Autodesk Fusion 360 part; units mm, degrees
(part 7 of 40)
  line L2812 (187.5144, 92.3152) -> (187.4885, 92.1609) construction
  line L2813 (187.4885, 92.1609) -> (187.4646, 92.006) construction
  line L2814 (187.4646, 92.006) -> (187.4423, 91.8506) construction
  line L2815 (187.4423, 91.8506) -> (187.4215, 91.6948) construction
  line L2816 (187.4215, 91.6948) -> (187.4019, 91.5386) construction
  line L2817 (187.4019, 91.5386) -> (187.3835, 91.3821) construction
  line L2818 (187.3835, 91.3821) -> (187.3662, 91.2253) construction
  line L2819 (187.3662, 91.2253) -> (187.3502, 91.0682) construction
  line L2820 (187.3502, 91.0682) -> (187.3355, 90.9107) construction
  line L2821 (187.3355, 90.9107) -> (187.3222, 90.7529) construction
  line L2822 (187.3222, 90.7529) -> (187.3102, 90.5947) construction
  line L2823 (187.3102, 90.5947) -> (187.2995, 90.4362) construction
  line L2824 (187.2995, 90.4362) -> (187.29, 90.2774) construction
  line L2825 (187.29, 90.2774) -> (187.2816, 90.1183) construction
  line L2826 (187.2816, 90.1183) -> (187.2743, 89.9589) construction
  line L2827 (187.2743, 89.9589) -> (187.2682, 89.7993) construction
  line L2828 (187.2682, 89.7993) -> (187.2631, 89.6395) construction
  line L2829 (187.2631, 89.6395) -> (187.2591, 89.4794) construction
  line L2830 (187.2591, 89.4794) -> (187.2563, 89.3191) construction
  line L2831 (187.2563, 89.3191) -> (187.2544, 89.1585) construction
  line L2832 (187.2544, 89.1585) -> (187.2537, 88.9977) construction
  line L2833 (187.2537, 88.9977) -> (187.254, 88.8367) construction
  line L2834 (187.254, 88.8367) -> (187.2554, 88.6755) construction
  line L2835 (187.2554, 88.6755) -> (187.2578, 88.5141) construction
  line L2836 (187.2578, 88.5141) -> (187.2612, 88.3525) construction
  line L2837 (187.2612, 88.3525) -> (187.2655, 88.1907) construction
  line L2838 (187.2655, 88.1907) -> (187.2709, 88.0288) construction
  line L2839 (187.2709, 88.0288) -> (187.2772, 87.8666) construction
  line L2840 (187.2772, 87.8666) -> (187.2845, 87.7043) construction
  line L2841 (187.2845, 87.7043) -> (187.2928, 87.5419) construction
  line L2842 (187.2928, 87.5419) -> (187.302, 87.3793) construction
  line L2843 (187.302, 87.3793) -> (187.3121, 87.2165) construction
  line L2844 (187.3121, 87.2165) -> (187.3232, 87.0536) construction
  line L2845 (187.3232, 87.0536) -> (187.3353, 86.8905) construction
  line L2846 (187.3353, 86.8905) -> (187.3482, 86.7273) construction
  line L2847 (187.3482, 86.7273) -> (187.362, 86.564) construction
  line L2848 (187.362, 86.564) -> (187.3768, 86.4005) construction
  line L2849 (187.3768, 86.4005) -> (187.3924, 86.2369) construction
  line L2850 (187.3924, 86.2369) -> (187.409, 86.0732) construction
  line L2851 (187.409, 86.0732) -> (187.4264, 85.9094) construction
  line L2852 (187.4264, 85.9094) -> (187.4447, 85.7455) construction
  line L2853 (187.4447, 85.7455) -> (187.4639, 85.5815) construction
  line L2854 (187.4639, 85.5815) -> (187.484, 85.4174) construction
  line L2855 (187.484, 85.4174) -> (187.5049, 85.2532) construction
  line L2856 (187.5049, 85.2532) -> (187.5266, 85.0889) construction
  line L2857 (187.5266, 85.0889) -> (187.5492, 84.9245) construction
  line L2858 (187.5492, 84.9245) -> (187.5727, 84.76) construction
  line L2859 (187.5727, 84.76) -> (187.597, 84.5954) construction
  line L2860 (187.597, 84.5954) -> (187.6222, 84.4308) construction
  line L2861 (187.6222, 84.4308) -> (187.6481, 84.266) construction
  line L2862 (187.6481, 84.266) -> (187.6749, 84.1013) construction
  line L2863 (187.6749, 84.1013) -> (187.7026, 83.9364) construction
  line L2864 (187.7026, 83.9364) -> (187.731, 83.7715) construction
  line L2865 (187.731, 83.7715) -> (187.7602, 83.6065) construction
  line L2866 (187.7602, 83.6065) -> (187.7903, 83.4415) construction
  line L2867 (187.7903, 83.4415) -> (187.8212, 83.2764) construction
  line L2868 (187.8212, 83.2764) -> (187.8528, 83.1113) construction
  line L2869 (187.8528, 83.1113) -> (187.8788, 82.9792) construction
  line L2870 (187.8788, 82.9792) -> (187.8986, 82.8801) construction
  line L2871 (187.8986, 82.8801) -> (187.912, 82.814) construction
  line L2872 (187.912, 82.814) -> (187.9188, 82.7809) construction
  arc A97 (187.9188, 82.7809) -> (192.2105, 81.3864) centre (212.132, 150) ccw
  arc A98 (187.9188, 82.7809) -> (192.2105, 81.3864) centre (212.132, 150) ccw
  line L2873 (256.7226, 110.7517) -> (257.9473, 109.6737)
  line L2874 (256.7226, 110.7517) -> (257.9473, 109.6737)
  arc A99 (269.1057, 157.2806) -> (268.567, 160.6816) centre (212.132, 150) ccw
  arc A100 (269.1057, 157.2806) -> (268.567, 160.6816) centre (212.132, 150) ccw
  arc A101 (256.7226, 110.7517) -> (253.9452, 110.6216) centre (255.4012, 109.2504) ccw
  arc A102 (256.7226, 110.7517) -> (253.9452, 110.6216) centre (255.4012, 109.2504) ccw
  arc A103 (251.5104, 108.1868) -> (253.9452, 110.6216) centre (212.132, 150) ccw
  arc A104 (251.5104, 108.1868) -> (253.9452, 110.6216) centre (212.132, 150) ccw
  spline S38 degree 5 poles (257.9473, 109.6737) (257.9705, 109.6533) (258.0174, 109.6132) (258.0893, 109.5549) (258.188, 109.4808) (258.3153, 109.3934) (258.4455, 109.3096) (258.5774, 109.228) (258.7102, 109.1476) (258.8437, 109.068) (258.9778, 108.9893) (259.1127, 108.9117) (259.2488, 108.8358) (259.3863, 108.7617) (259.525, 108.6894) (259.6649, 108.6187) (259.8058, 108.5496) (259.9476, 108.4816) (260.0901, 108.4147) (260.2332, 108.3488) (260.377, 108.284) (260.5215, 108.2202) (260.6667, 108.1576) (260.8127, 108.0961) (260.9594, 108.0358) (261.1069, 107.9766) (261.255, 107.9185) (261.4037, 107.8614) (261.553, 107.8053) (261.7029, 107.7501) (261.8534, 107.6959) (262.0044, 107.6426) (262.156, 107.5903) (262.3081, 107.539) (262.4608, 107.4886) (262.614, 107.4392) (262.7678, 107.3906) (262.922, 107.343) (263.0767, 107.2963) (263.2319, 107.2505) (263.3876, 107.2055) (263.5438, 107.1614) (263.7004, 107.1182) (263.8575, 107.0759) (264.015, 107.0344) (264.1729, 106.9937) (264.3313, 106.9539) (264.4901, 106.915) (264.6493, 106.8769) (264.8089, 106.8396) (264.9689, 106.8031) (265.1293, 106.7674) (265.2901, 106.7326) (265.4513, 106.6985) (265.6129, 106.6653) (265.7748, 106.6328) (265.9371, 106.6012) (266.0997, 106.5703) (266.2627, 106.5403) (266.426, 106.511) (266.5897, 106.4825) (266.7537, 106.4547) (266.9181, 106.4277) (267.0828, 106.4016) (267.2478, 106.3761) (267.4131, 106.3514) (267.5787, 106.3275) (267.7446, 106.3044) (267.9109, 106.282) (268.0774, 106.2603) (268.2442, 106.2394) (268.3779, 106.2233) (268.4783, 106.2115) (268.5453, 106.2038) (268.5789, 106.2) knots 0 0 0 0 0 0 0.01428571 0.02857143 0.04285714 0.05714286 0.07142857 0.08571429 0.1 0.11428571 0.12857143 0.14285714 0.15714286 0.17142857 0.18571429 0.2 0.21428571 0.22857143 0.24285714 0.25714286 0.27142857 0.28571429 0.3 0.31428571 0.32857143 0.34285714 0.35714286 0.37142857 0.38571429 0.4 0.41428571 0.42857143 0.44285714 0.45714286 0.47142857 0.48571429 0.5 0.51428571 0.52857143 0.54285714 0.55714286 0.57142857 0.58571429 0.6 0.61428571 0.62857143 0.64285714 0.65714286 0.67142857 0.68571429 0.7 0.71428571 0.72857143 0.74285714 0.75714286 0.77142857 0.78571429 0.8 0.81428571 0.82857143 0.84285714 0.85714286 0.87142857 0.88571429 0.9 0.91428571 0.92857143 0.94285714 0.95714286 0.97142857 0.98571429 1 1 1 1 1 1
  line L2875 (257.9473, 109.6737) -> (257.9705, 109.6533) construction
  line L2876 (257.9705, 109.6533) -> (258.0174, 109.6132) construction
  line L2877 (258.0174, 109.6132) -> (258.0893, 109.5549) construction
  line L2878 (258.0893, 109.5549) -> (258.188, 109.4808) construction
  line L2879 (258.188, 109.4808) -> (258.3153, 109.3934) construction
  line L2880 (258.3153, 109.3934) -> (258.4455, 109.3096) construction
  line L2881 (258.4455, 109.3096) -> (258.5774, 109.228) construction
  line L2882 (258.5774, 109.228) -> (258.7102, 109.1476) construction
  line L2883 (258.7102, 109.1476) -> (258.8437, 109.068) construction
  line L2884 (258.8437, 109.068) -> (258.9778, 108.9893) construction
  line L2885 (258.9778, 108.9893) -> (259.1127, 108.9117) construction
  line L2886 (259.1127, 108.9117) -> (259.2488, 108.8358) construction
  line L2887 (259.2488, 108.8358) -> (259.3863, 108.7617) construction
  line L2888 (259.3863, 108.7617) -> (259.525, 108.6894) construction
  line L2889 (259.525, 108.6894) -> (259.6649, 108.6187) construction
  line L2890 (259.6649, 108.6187) -> (259.8058, 108.5496) construction
  line L2891 (259.8058, 108.5496) -> (259.9476, 108.4816) construction
  line L2892 (259.9476, 108.4816) -> (260.0901, 108.4147) construction
  line L2893 (260.0901, 108.4147) -> (260.2332, 108.3488) construction
  line L2894 (260.2332, 108.3488) -> (260.377, 108.284) construction
  line L2895 (260.377, 108.284) -> (260.5215, 108.2202) construction
  line L2896 (260.5215, 108.2202) -> (260.6667, 108.1576) construction
  line L2897 (260.6667, 108.1576) -> (260.8127, 108.0961) construction
  line L2898 (260.8127, 108.0961) -> (260.9594, 108.0358) construction
  line L2899 (260.9594, 108.0358) -> (261.1069, 107.9766) construction
  line L2900 (261.1069, 107.9766) -> (261.255, 107.9185) construction
  line L2901 (261.255, 107.9185) -> (261.4037, 107.8614) construction
  line L2902 (261.4037, 107.8614) -> (261.553, 107.8053) construction
  line L2903 (261.553, 107.8053) -> (261.7029, 107.7501) construction
  line L2904 (261.7029, 107.7501) -> (261.8534, 107.6959) construction
  line L2905 (261.8534, 107.6959) -> (262.0044, 107.6426) construction
  line L2906 (262.0044, 107.6426) -> (262.156, 107.5903) construction
  line L2907 (262.156, 107.5903) -> (262.3081, 107.539) construction
  line L2908 (262.3081, 107.539) -> (262.4608, 107.4886) construction
  line L2909 (262.4608, 107.4886) -> (262.614, 107.4392) construction
  line L2910 (262.614, 107.4392) -> (262.7678, 107.3906) construction
  line L2911 (262.7678, 107.3906) -> (262.922, 107.343) construction
  line L2912 (262.922, 107.343) -> (263.0767, 107.2963) construction
  line L2913 (263.0767, 107.2963) -> (263.2319, 107.2505) construction
  line L2914 (263.2319, 107.2505) -> (263.3876, 107.2055) construction
  line L2915 (263.3876, 107.2055) -> (263.5438, 107.1614) construction
  line L2916 (263.5438, 107.1614) -> (263.7004, 107.1182) construction
  line L2917 (263.7004, 107.1182) -> (263.8575, 107.0759) construction
  line L2918 (263.8575, 107.0759) -> (264.015, 107.0344) construction
  line L2919 (264.015, 107.0344) -> (264.1729, 106.9937) construction
  line L2920 (264.1729, 106.9937) -> (264.3313, 106.9539) construction
  line L2921 (264.3313, 106.9539) -> (264.4901, 106.915) construction
  line L2922 (264.4901, 106.915) -> (264.6493, 106.8769) construction
  line L2923 (264.6493, 106.8769) -> (264.8089, 106.8396) construction
  line L2924 (264.8089, 106.8396) -> (264.9689, 106.8031) construction
  line L2925 (264.9689, 106.8031) -> (265.1293, 106.7674) construction
  line L2926 (265.1293, 106.7674) -> (265.2901, 106.7326) construction
  line L2927 (265.2901, 106.7326) -> (265.4513, 106.6985) construction
  line L2928 (265.4513, 106.6985) -> (265.6129, 106.6653) construction
  line L2929 (265.6129, 106.6653) -> (265.7748, 106.6328) construction
  line L2930 (265.7748, 106.6328) -> (265.9371, 106.6012) construction
  line L2931 (265.9371, 106.6012) -> (266.0997, 106.5703) construction
  line L2932 (266.0997, 106.5703) -> (266.2627, 106.5403) construction
  line L2933 (266.2627, 106.5403) -> (266.426, 106.511) construction
  line L2934 (266.426, 106.511) -> (266.5897, 106.4825) construction
  line L2935 (266.5897, 106.4825) -> (266.7537, 106.4547) construction
  line L2936 (266.7537, 106.4547) -> (266.9181, 106.4277) construction
  line L2937 (266.9181, 106.4277) -> (267.0828, 106.4016) construction
  line L2938 (267.0828, 106.4016) -> (267.2478, 106.3761) construction
  line L2939 (267.2478, 106.3761) -> (267.4131, 106.3514) construction
  line L2940 (267.4131, 106.3514) -> (267.5787, 106.3275) construction
  line L2941 (267.5787, 106.3275) -> (267.7446, 106.3044) construction
  line L2942 (267.7446, 106.3044) -> (267.9109, 106.282) construction
  line L2943 (267.9109, 106.282) -> (268.0774, 106.2603) construction
  line L2944 (268.0774, 106.2603) -> (268.2442, 106.2394) construction
  line L2945 (268.2442, 106.2394) -> (268.3779, 106.2233) construction
  line L2946 (268.3779, 106.2233) -> (268.4783, 106.2115) construction
  line L2947 (268.4783, 106.2115) -> (268.5453, 106.2038) construction
  line L2948 (268.5453, 106.2038) -> (268.5789, 106.2) construction
  line L2949 (271.2762, 155.5428) -> (272.9005, 155.6951)
  spline S39 degree 5 poles (257.9473, 109.6737) (257.9705, 109.6533) (258.0174, 109.6132) (258.0893, 109.5549) (258.188, 109.4808) (258.3153, 109.3934) (258.4455, 109.3096) (258.5774, 109.228) (258.7102, 109.1476) (258.8437, 109.068) (258.9778, 108.9893) (259.1127, 108.9117) (259.2488, 108.8358) (259.3863, 108.7617) (259.525, 108.6894) (259.6649, 108.6187) (259.8058, 108.5496) (259.9476, 108.4816) (260.0901, 108.4147) (260.2332, 108.3488) (260.377, 108.284) (260.5215, 108.2202) (260.6667, 108.1576) (260.8127, 108.0961) (260.9594, 108.0358) (261.1069, 107.9766) (261.255, 107.9185) (261.4037, 107.8614) (261.553, 107.8053) (261.7029, 107.7501) (261.8534, 107.6959) (262.0044, 107.6426) (262.156, 107.5903) (262.3081, 107.539) (262.4608, 107.4886) (262.614, 107.4392) (262.7678, 107.3906) (262.922, 107.343) (263.0767, 107.2963) (263.2319, 107.2505) (263.3876, 107.2055) (263.5438, 107.1614) (263.7004, 107.1182) (263.8575, 107.0759) (264.015, 107.0344) (264.1729, 106.9937) (264.3313, 106.9539) (264.4901, 106.915) (264.6493, 106.8769) (264.8089, 106.8396) (264.9689, 106.8031) (265.1293, 106.7674) (265.2901, 106.7326) (265.4513, 106.6985) (265.6129, 106.6653) (265.7748, 106.6328) (265.9371, 106.6012) (266.0997, 106.5703) (266.2627, 106.5403) (266.426, 106.511) (266.5897, 106.4825) (266.7537, 106.4547) (266.9181, 106.4277) (267.0828, 106.4016) (267.2478, 106.3761) (267.4131, 106.3514) (267.5787, 106.3275) (267.7446, 106.3044) (267.9109, 106.282) (268.0774, 106.2603) (268.2442, 106.2394) (268.3779, 106.2233) (268.4783, 106.2115) (268.5453, 106.2038) (268.5789, 106.2) knots 0 0 0 0 0 0 0.01428571 0.02857143 0.04285714 0.05714286 0.07142857 0.08571429 0.1 0.11428571 0.12857143 0.14285714 0.15714286 0.17142857 0.18571429 0.2 0.21428571 0.22857143 0.24285714 0.25714286 0.27142857 0.28571429 0.3 0.31428571 0.32857143 0.34285714 0.35714286 0.37142857 0.38571429 0.4 0.41428571 0.42857143 0.44285714 0.45714286 0.47142857 0.48571429 0.5 0.51428571 0.52857143 0.54285714 0.55714286 0.57142857 0.58571429 0.6 0.61428571 0.62857143 0.64285714 0.65714286 0.67142857 0.68571429 0.7 0.71428571 0.72857143 0.74285714 0.75714286 0.77142857 0.78571429 0.8 0.81428571 0.82857143 0.84285714 0.85714286 0.87142857 0.88571429 0.9 0.91428571 0.92857143 0.94285714 0.95714286 0.97142857 0.98571429 1 1 1 1 1 1
  line L2950 (257.9473, 109.6737) -> (257.9705, 109.6533) construction
  line L2951 (257.9705, 109.6533) -> (258.0174, 109.6132) construction
  line L2952 (258.0174, 109.6132) -> (258.0893, 109.5549) construction
  line L2953 (258.0893, 109.5549) -> (258.188, 109.4808) construction
  line L2954 (258.188, 109.4808) -> (258.3153, 109.3934) construction
  line L2955 (258.3153, 109.3934) -> (258.4455, 109.3096) construction
  line L2956 (258.4455, 109.3096) -> (258.5774, 109.228) construction
  line L2957 (258.5774, 109.228) -> (258.7102, 109.1476) construction
  line L2958 (258.7102, 109.1476) -> (258.8437, 109.068) construction
  line L2959 (258.8437, 109.068) -> (258.9778, 108.9893) construction
  line L2960 (258.9778, 108.9893) -> (259.1127, 108.9117) construction
  line L2961 (259.1127, 108.9117) -> (259.2488, 108.8358) construction
  line L2962 (259.2488, 108.8358) -> (259.3863, 108.7617) construction
  line L2963 (259.3863, 108.7617) -> (259.525, 108.6894) construction
  line L2964 (259.525, 108.6894) -> (259.6649, 108.6187) construction
  line L2965 (259.6649, 108.6187) -> (259.8058, 108.5496) construction
  line L2966 (259.8058, 108.5496) -> (259.9476, 108.4816) construction
  line L2967 (259.9476, 108.4816) -> (260.0901, 108.4147) construction
  line L2968 (260.0901, 108.4147) -> (260.2332, 108.3488) construction
  line L2969 (260.2332, 108.3488) -> (260.377, 108.284) construction
  line L2970 (260.377, 108.284) -> (260.5215, 108.2202) construction
  line L2971 (260.5215, 108.2202) -> (260.6667, 108.1576) construction
  line L2972 (260.6667, 108.1576) -> (260.8127, 108.0961) construction
  line L2973 (260.8127, 108.0961) -> (260.9594, 108.0358) construction
  line L2974 (260.9594, 108.0358) -> (261.1069, 107.9766) construction
  line L2975 (261.1069, 107.9766) -> (261.255, 107.9185) construction
  line L2976 (261.255, 107.9185) -> (261.4037, 107.8614) construction
  line L2977 (261.4037, 107.8614) -> (261.553, 107.8053) construction
  line L2978 (261.553, 107.8053) -> (261.7029, 107.7501) construction
  line L2979 (261.7029, 107.7501) -> (261.8534, 107.6959) construction
  line L2980 (261.8534, 107.6959) -> (262.0044, 107.6426) construction
  line L2981 (262.0044, 107.6426) -> (262.156, 107.5903) construction
  line L2982 (262.156, 107.5903) -> (262.3081, 107.539) construction
  line L2983 (262.3081, 107.539) -> (262.4608, 107.4886) construction
  line L2984 (262.4608, 107.4886) -> (262.614, 107.4392) construction
  line L2985 (262.614, 107.4392) -> (262.7678, 107.3906) construction
  line L2986 (262.7678, 107.3906) -> (262.922, 107.343) construction
  line L2987 (262.922, 107.343) -> (263.0767, 107.2963) construction
  line L2988 (263.0767, 107.2963) -> (263.2319, 107.2505) construction
  line L2989 (263.2319, 107.2505) -> (263.3876, 107.2055) construction
  line L2990 (263.3876, 107.2055) -> (263.5438, 107.1614) construction
  line L2991 (263.5438, 107.1614) -> (263.7004, 107.1182) construction
  line L2992 (263.7004, 107.1182) -> (263.8575, 107.0759) construction
  line L2993 (263.8575, 107.0759) -> (264.015, 107.0344) construction
  line L2994 (264.015, 107.0344) -> (264.1729, 106.9937) construction
  line L2995 (264.1729, 106.9937) -> (264.3313, 106.9539) construction
  line L2996 (264.3313, 106.9539) -> (264.4901, 106.915) construction
  line L2997 (264.4901, 106.915) -> (264.6493, 106.8769) construction
  line L2998 (264.6493, 106.8769) -> (264.8089, 106.8396) construction
  line L2999 (264.8089, 106.8396) -> (264.9689, 106.8031) construction
  line L3000 (264.9689, 106.8031) -> (265.1293, 106.7674) construction
  line L3001 (265.1293, 106.7674) -> (265.2901, 106.7326) construction
  line L3002 (265.2901, 106.7326) -> (265.4513, 106.6985) construction
  line L3003 (265.4513, 106.6985) -> (265.6129, 106.6653) construction
  line L3004 (265.6129, 106.6653) -> (265.7748, 106.6328) construction
  line L3005 (265.7748, 106.6328) -> (265.9371, 106.6012) construction
  line L3006 (265.9371, 106.6012) -> (266.0997, 106.5703) construction
  line L3007 (266.0997, 106.5703) -> (266.2627, 106.5403) construction
  line L3008 (266.2627, 106.5403) -> (266.426, 106.511) construction
  line L3009 (266.426, 106.511) -> (266.5897, 106.4825) construction
  line L3010 (266.5897, 106.4825) -> (266.7537, 106.4547) construction
  line L3011 (266.7537, 106.4547) -> (266.9181, 106.4277) construction
  line L3012 (266.9181, 106.4277) -> (267.0828, 106.4016) construction
  line L3013 (267.0828, 106.4016) -> (267.2478, 106.3761) construction
  line L3014 (267.2478, 106.3761) -> (267.4131, 106.3514) construction
  line L3015 (267.4131, 106.3514) -> (267.5787, 106.3275) construction
  line L3016 (267.5787, 106.3275) -> (267.7446, 106.3044) construction
  line L3017 (267.7446, 106.3044) -> (267.9109, 106.282) construction
  line L3018 (267.9109, 106.282) -> (268.0774, 106.2603) construction
  line L3019 (268.0774, 106.2603) -> (268.2442, 106.2394) construction
  line L3020 (268.2442, 106.2394) -> (268.3779, 106.2233) construction
  line L3021 (268.3779, 106.2233) -> (268.4783, 106.2115) construction
  line L3022 (268.4783, 106.2115) -> (268.5453, 106.2038) construction
  line L3023 (268.5453, 106.2038) -> (268.5789, 106.2) construction
  spline S40 degree 5 poles (271.6862, 136.6378) (271.7163, 136.631) (271.7764, 136.6167) (271.8658, 136.5929) (271.9837, 136.5565) (272.1293, 136.5049) (272.2736, 136.4489) (272.4172, 136.3901) (272.5603, 136.3299) (272.7031, 136.2687) (272.8456, 136.2065) (272.9877, 136.1429) (273.1291, 136.0774) (273.2699, 136.0098) (273.4099, 135.94) (273.5493, 135.8684) (273.6881, 135.795) (273.8264, 135.7203) (273.9642, 135.6443) (274.1017, 135.5673) (274.2387, 135.4891) (274.3752, 135.4096) (274.5112, 135.3289) (274.6468, 135.247) (274.7818, 135.1637) (274.9163, 135.0792) (275.0504, 134.9936) (275.184, 134.9068) (275.3172, 134.819) (275.45, 134.7302) (275.5823, 134.6403) (275.7141, 134.5494) (275.8455, 134.4575) (275.9765, 134.3646) (276.107, 134.2707) (276.237, 134.1758) (276.3666, 134.08) (276.4958, 133.9832) (276.6246, 133.8854) (276.7529, 133.7868) (276.8808, 133.6873) (277.0082, 133.5869) (277.1352, 133.4856) (277.2618, 133.3834) (277.388, 133.2804) (277.5137, 133.1765) (277.639, 133.0717) (277.7638, 132.9662) (277.8882, 132.8598) (278.0122, 132.7526) (278.1358, 132.6445) (278.2589, 132.5357) (278.3817, 132.4261) (278.5039, 132.3158) (278.6258, 132.2046) (278.7472, 132.0927) (278.8682, 131.98) (278.9888, 131.8665) (279.1089, 131.7523) (279.2286, 131.6374) (279.3479, 131.5218) (279.4667, 131.4054) (279.5851, 131.2882) (279.7031, 131.1704) (279.8207, 131.0519) (279.9378, 130.9326) (280.0545, 130.8127) (280.1708, 130.6921) (280.2866, 130.5707) (280.402, 130.4488) (280.517, 130.3261) (280.6087, 130.2274) (280.6772, 130.1531) (280.7228, 130.1034) (280.7456, 130.0785) knots 0 0 0 0 0 0 0.01428571 0.02857143 0.04285714 0.05714286 0.07142857 0.08571429 0.1 0.11428571 0.12857143 0.14285714 0.15714286 0.17142857 0.18571429 0.2 0.21428571 0.22857143 0.24285714 0.25714286 0.27142857 0.28571429 0.3 0.31428571 0.32857143 0.34285714 0.35714286 0.37142857 0.38571429 0.4 0.41428571 0.42857143 0.44285714 0.45714286 0.47142857 0.48571429 0.5 0.51428571 0.52857143 0.54285714 0.55714286 0.57142857 0.58571429 0.6 0.61428571 0.62857143 0.64285714 0.65714286 0.67142857 0.68571429 0.7 0.71428571 0.72857143 0.74285714 0.75714286 0.77142857 0.78571429 0.8 0.81428571 0.82857143 0.84285714 0.85714286 0.87142857 0.88571429 0.9 0.91428571 0.92857143 0.94285714 0.95714286 0.97142857 0.98571429 1 1 1 1 1 1
  line L3024 (271.6862, 136.6378) -> (271.7163, 136.631) construction
  line L3025 (271.7163, 136.631) -> (271.7764, 136.6167) construction
  line L3026 (271.7764, 136.6167) -> (271.8658, 136.5929) construction
  line L3027 (271.8658, 136.5929) -> (271.9837, 136.5565) construction
  line L3028 (271.9837, 136.5565) -> (272.1293, 136.5049) construction
  line L3029 (272.1293, 136.5049) -> (272.2736, 136.4489) construction
  line L3030 (272.2736, 136.4489) -> (272.4172, 136.3901) construction
  line L3031 (272.4172, 136.3901) -> (272.5603, 136.3299) construction
  line L3032 (272.5603, 136.3299) -> (272.7031, 136.2687) construction
  line L3033 (272.7031, 136.2687) -> (272.8456, 136.2065) construction
  line L3034 (272.8456, 136.2065) -> (272.9877, 136.1429) construction
  line L3035 (272.9877, 136.1429) -> (273.1291, 136.0774) construction
  line L3036 (273.1291, 136.0774) -> (273.2699, 136.0098) construction
  line L3037 (273.2699, 136.0098) -> (273.4099, 135.94) construction
  line L3038 (273.4099, 135.94) -> (273.5493, 135.8684) construction
  line L3039 (273.5493, 135.8684) -> (273.6881, 135.795) construction
  line L3040 (273.6881, 135.795) -> (273.8264, 135.7203) construction
  line L3041 (273.8264, 135.7203) -> (273.9642, 135.6443) construction
  line L3042 (273.9642, 135.6443) -> (274.1017, 135.5673) construction
  line L3043 (274.1017, 135.5673) -> (274.2387, 135.4891) construction
  line L3044 (274.2387, 135.4891) -> (274.3752, 135.4096) construction
  line L3045 (274.3752, 135.4096) -> (274.5112, 135.3289) construction
  line L3046 (274.5112, 135.3289) -> (274.6468, 135.247) construction
  line L3047 (274.6468, 135.247) -> (274.7818, 135.1637) construction
  line L3048 (274.7818, 135.1637) -> (274.9163, 135.0792) construction
  line L3049 (274.9163, 135.0792) -> (275.0504, 134.9936) construction
  line L3050 (275.0504, 134.9936) -> (275.184, 134.9068) construction
  line L3051 (275.184, 134.9068) -> (275.3172, 134.819) construction
  line L3052 (275.3172, 134.819) -> (275.45, 134.7302) construction
  line L3053 (275.45, 134.7302) -> (275.5823, 134.6403) construction
  line L3054 (275.5823, 134.6403) -> (275.7141, 134.5494) construction
  line L3055 (275.7141, 134.5494) -> (275.8455, 134.4575) construction
  line L3056 (275.8455, 134.4575) -> (275.9765, 134.3646) construction
  line L3057 (275.9765, 134.3646) -> (276.107, 134.2707) construction
  line L3058 (276.107, 134.2707) -> (276.237, 134.1758) construction
  line L3059 (276.237, 134.1758) -> (276.3666, 134.08) construction
  line L3060 (276.3666, 134.08) -> (276.4958, 133.9832) construction
  line L3061 (276.4958, 133.9832) -> (276.6246, 133.8854) construction
  line L3062 (276.6246, 133.8854) -> (276.7529, 133.7868) construction
  line L3063 (276.7529, 133.7868) -> (276.8808, 133.6873) construction
  line L3064 (276.8808, 133.6873) -> (277.0082, 133.5869) construction
  line L3065 (277.0082, 133.5869) -> (277.1352, 133.4856) construction
  line L3066 (277.1352, 133.4856) -> (277.2618, 133.3834) construction
  line L3067 (277.2618, 133.3834) -> (277.388, 133.2804) construction
  line L3068 (277.388, 133.2804) -> (277.5137, 133.1765) construction
  line L3069 (277.5137, 133.1765) -> (277.639, 133.0717) construction
  line L3070 (277.639, 133.0717) -> (277.7638, 132.9662) construction
  line L3071 (277.7638, 132.9662) -> (277.8882, 132.8598) construction
  line L3072 (277.8882, 132.8598) -> (278.0122, 132.7526) construction
  line L3073 (278.0122, 132.7526) -> (278.1358, 132.6445) construction
  line L3074 (278.1358, 132.6445) -> (278.2589, 132.5357) construction
  line L3075 (278.2589, 132.5357) -> (278.3817, 132.4261) construction
  line L3076 (278.3817, 132.4261) -> (278.5039, 132.3158) construction
  line L3077 (278.5039, 132.3158) -> (278.6258, 132.2046) construction
  line L3078 (278.6258, 132.2046) -> (278.7472, 132.0927) construction
  line L3079 (278.7472, 132.0927) -> (278.8682, 131.98) construction
  line L3080 (278.8682, 131.98) -> (278.9888, 131.8665) construction
  line L3081 (278.9888, 131.8665) -> (279.1089, 131.7523) construction
  line L3082 (279.1089, 131.7523) -> (279.2286, 131.6374) construction
  line L3083 (279.2286, 131.6374) -> (279.3479, 131.5218) construction
  line L3084 (279.3479, 131.5218) -> (279.4667, 131.4054) construction
  line L3085 (279.4667, 131.4054) -> (279.5851, 131.2882) construction
  line L3086 (279.5851, 131.2882) -> (279.7031, 131.1704) construction
  line L3087 (279.7031, 131.1704) -> (279.8207, 131.0519) construction
  line L3088 (279.8207, 131.0519) -> (279.9378, 130.9326) construction
  line L3089 (279.9378, 130.9326) -> (280.0545, 130.8127) construction
  line L3090 (280.0545, 130.8127) -> (280.1708, 130.6921) construction
  line L3091 (280.1708, 130.6921) -> (280.2866, 130.5707) construction
  line L3092 (280.2866, 130.5707) -> (280.402, 130.4488) construction
  line L3093 (280.402, 130.4488) -> (280.517, 130.3261) construction
  line L3094 (280.517, 130.3261) -> (280.6087, 130.2274) construction
  line L3095 (280.6087, 130.2274) -> (280.6772, 130.1531) construction
  line L3096 (280.6772, 130.1531) -> (280.7228, 130.1034) construction
  line L3097 (280.7228, 130.1034) -> (280.7456, 130.0785) construction
  spline S41 degree 5 poles (271.6862, 136.6378) (271.7163, 136.631) (271.7764, 136.6167) (271.8658, 136.5929) (271.9837, 136.5565) (272.1293, 136.5049) (272.2736, 136.4489) (272.4172, 136.3901) (272.5603, 136.3299) (272.7031, 136.2687) (272.8456, 136.2065) (272.9877, 136.1429) (273.1291, 136.0774) (273.2699, 136.0098) (273.4099, 135.94) (273.5493, 135.8684) (273.6881, 135.795) (273.8264, 135.7203) (273.9642, 135.6443) (274.1017, 135.5673) (274.2387, 135.4891) (274.3752, 135.4096) (274.5112, 135.3289) (274.6468, 135.247) (274.7818, 135.1637) (274.9163, 135.0792) (275.0504, 134.9936) (275.184, 134.9068) (275.3172, 134.819) (275.45, 134.7302) (275.5823, 134.6403) (275.7141, 134.5494) (275.8455, 134.4575) (275.9765, 134.3646) (276.107, 134.2707) (276.237, 134.1758) (276.3666, 134.08) (276.4958, 133.9832) (276.6246, 133.8854) (276.7529, 133.7868) (276.8808, 133.6873) (277.0082, 133.5869) (277.1352, 133.4856) (277.2618, 133.3834) (277.388, 133.2804) (277.5137, 133.1765) (277.639, 133.0717) (277.7638, 132.9662) (277.8882, 132.8598) (278.0122, 132.7526) (278.1358, 132.6445) (278.2589, 132.5357) (278.3817, 132.4261) (278.5039, 132.3158) (278.6258, 132.2046) (278.7472, 132.0927) (278.8682, 131.98) (278.9888, 131.8665) (279.1089, 131.7523) (279.2286, 131.6374) (279.3479, 131.5218) (279.4667, 131.4054) (279.5851, 131.2882) (279.7031, 131.1704) (279.8207, 131.0519) (279.9378, 130.9326) (280.0545, 130.8127) (280.1708, 130.6921) (280.2866, 130.5707) (280.402, 130.4488) (280.517, 130.3261) (280.6087, 130.2274) (280.6772, 130.1531) (280.7228, 130.1034) (280.7456, 130.0785) knots 0 0 0 0 0 0 0.01428571 0.02857143 0.04285714 0.05714286 0.07142857 0.08571429 0.1 0.11428571 0.12857143 0.14285714 0.15714286 0.17142857 0.18571429 0.2 0.21428571 0.22857143 0.24285714 0.25714286 0.27142857 0.28571429 0.3 0.31428571 0.32857143 0.34285714 0.35714286 0.37142857 0.38571429 0.4 0.41428571 0.42857143 0.44285714 0.45714286 0.47142857 0.48571429 0.5 0.51428571 0.52857143 0.54285714 0.55714286 0.57142857 0.58571429 0.6 0.61428571 0.62857143 0.64285714 0.65714286 0.67142857 0.68571429 0.7 0.71428571 0.72857143 0.74285714 0.75714286 0.77142857 0.78571429 0.8 0.81428571 0.82857143 0.84285714 0.85714286 0.87142857 0.88571429 0.9 0.91428571 0.92857143 0.94285714 0.95714286 0.97142857 0.98571429 1 1 1 1 1 1
  line L3098 (271.6862, 136.6378) -> (271.7163, 136.631) construction
  line L3099 (271.7163, 136.631) -> (271.7764, 136.6167) construction
  line L3100 (271.7764, 136.6167) -> (271.8658, 136.5929) construction
  line L3101 (271.8658, 136.5929) -> (271.9837, 136.5565) construction
  line L3102 (271.9837, 136.5565) -> (272.1293, 136.5049) construction
  line L3103 (272.1293, 136.5049) -> (272.2736, 136.4489) construction
  line L3104 (272.2736, 136.4489) -> (272.4172, 136.3901) construction
  line L3105 (272.4172, 136.3901) -> (272.5603, 136.3299) construction
  line L3106 (272.5603, 136.3299) -> (272.7031, 136.2687) construction
  line L3107 (272.7031, 136.2687) -> (272.8456, 136.2065) construction
  line L3108 (272.8456, 136.2065) -> (272.9877, 136.1429) construction
  line L3109 (272.9877, 136.1429) -> (273.1291, 136.0774) construction
  line L3110 (273.1291, 136.0774) -> (273.2699, 136.0098) construction
  line L3111 (273.2699, 136.0098) -> (273.4099, 135.94) construction
  line L3112 (273.4099, 135.94) -> (273.5493, 135.8684) construction
  line L3113 (273.5493, 135.8684) -> (273.6881, 135.795) construction
  line L3114 (273.6881, 135.795) -> (273.8264, 135.7203) construction
  line L3115 (273.8264, 135.7203) -> (273.9642, 135.6443) construction
  line L3116 (273.9642, 135.6443) -> (274.1017, 135.5673) construction
  line L3117 (274.1017, 135.5673) -> (274.2387, 135.4891) construction
  line L3118 (274.2387, 135.4891) -> (274.3752, 135.4096) construction
  line L3119 (274.3752, 135.4096) -> (274.5112, 135.3289) construction
  line L3120 (274.5112, 135.3289) -> (274.6468, 135.247) construction
  line L3121 (274.6468, 135.247) -> (274.7818, 135.1637) construction
  line L3122 (274.7818, 135.1637) -> (274.9163, 135.0792) construction
  line L3123 (274.9163, 135.0792) -> (275.0504, 134.9936) construction
  line L3124 (275.0504, 134.9936) -> (275.184, 134.9068) construction
  line L3125 (275.184, 134.9068) -> (275.3172, 134.819) construction
  line L3126 (275.3172, 134.819) -> (275.45, 134.7302) construction
  line L3127 (275.45, 134.7302) -> (275.5823, 134.6403) construction
  line L3128 (275.5823, 134.6403) -> (275.7141, 134.5494) construction
  line L3129 (275.7141, 134.5494) -> (275.8455, 134.4575) construction
  line L3130 (275.8455, 134.4575) -> (275.9765, 134.3646) construction
  line L3131 (275.9765, 134.3646) -> (276.107, 134.2707) construction
  line L3132 (276.107, 134.2707) -> (276.237, 134.1758) construction
  line L3133 (276.237, 134.1758) -> (276.3666, 134.08) construction
  line L3134 (276.3666, 134.08) -> (276.4958, 133.9832) construction
  line L3135 (276.4958, 133.9832) -> (276.6246, 133.8854) construction
  line L3136 (276.6246, 133.8854) -> (276.7529, 133.7868) construction
  line L3137 (276.7529, 133.7868) -> (276.8808, 133.6873) construction
  line L3138 (276.8808, 133.6873) -> (277.0082, 133.5869) construction
  line L3139 (277.0082, 133.5869) -> (277.1352, 133.4856) construction
  line L3140 (277.1352, 133.4856) -> (277.2618, 133.3834) construction
  line L3141 (277.2618, 133.3834) -> (277.388, 133.2804) construction
  line L3142 (277.388, 133.2804) -> (277.5137, 133.1765) construction
  line L3143 (277.5137, 133.1765) -> (277.639, 133.0717) construction
  line L3144 (277.639, 133.0717) -> (277.7638, 132.9662) construction
  line L3145 (277.7638, 132.9662) -> (277.8882, 132.8598) construction
  line L3146 (277.8882, 132.8598) -> (278.0122, 132.7526) construction
  line L3147 (278.0122, 132.7526) -> (278.1358, 132.6445) construction
  line L3148 (278.1358, 132.6445) -> (278.2589, 132.5357) construction
  line L3149 (278.2589, 132.5357) -> (278.3817, 132.4261) construction
  line L3150 (278.3817, 132.4261) -> (278.5039, 132.3158) construction
  line L3151 (278.5039, 132.3158) -> (278.6258, 132.2046) construction
  line L3152 (278.6258, 132.2046) -> (278.7472, 132.0927) construction
  line L3153 (278.7472, 132.0927) -> (278.8682, 131.98) construction
  line L3154 (278.8682, 131.98) -> (278.9888, 131.8665) construction
  line L3155 (278.9888, 131.8665) -> (279.1089, 131.7523) construction
  line L3156 (279.1089, 131.7523) -> (279.2286, 131.6374) construction
  line L3157 (279.2286, 131.6374) -> (279.3479, 131.5218) construction
  line L3158 (279.3479, 131.5218) -> (279.4667, 131.4054) construction
  line L3159 (279.4667, 131.4054) -> (279.5851, 131.2882) construction
  line L3160 (279.5851, 131.2882) -> (279.7031, 131.1704) construction
  line L3161 (279.7031, 131.1704) -> (279.8207, 131.0519) construction
  line L3162 (279.8207, 131.0519) -> (279.9378, 130.9326) construction
  line L3163 (279.9378, 130.9326) -> (280.0545, 130.8127) construction
  line L3164 (280.0545, 130.8127) -> (280.1708, 130.6921) construction
  line L3165 (280.1708, 130.6921) -> (280.2866, 130.5707) construction
  line L3166 (280.2866, 130.5707) -> (280.402, 130.4488) construction
  line L3167 (280.402, 130.4488) -> (280.517, 130.3261) construction
  line L3168 (280.517, 130.3261) -> (280.6087, 130.2274) construction
  line L3169 (280.6087, 130.2274) -> (280.6772, 130.1531) construction
  line L3170 (280.6772, 130.1531) -> (280.7228, 130.1034) construction
  line L3171 (280.7228, 130.1034) -> (280.7456, 130.0785) construction
  spline S42 degree 5 poles (187.9372, 206.0345) (187.9249, 206.0628) (187.9012, 206.1198) (187.868, 206.2062) (187.8281, 206.3229) (187.7842, 206.4711) (187.7447, 206.6208) (187.7079, 206.7714) (187.6725, 206.9226) (187.638, 207.0741) (187.6046, 207.226) (187.5726, 207.3783) (187.5424, 207.5312) (187.5144, 207.6848) (187.4885, 207.8391) (187.4646, 207.994) (187.4423, 208.1494) (187.4215, 208.3052) (187.4019, 208.4614) (187.3835, 208.6179) (187.3662, 208.7747) (187.3502, 208.9318) (187.3355, 209.0893) (187.3222, 209.2471) (187.3102, 209.4053) (187.2995, 209.5638) (187.29, 209.7226) (187.2816, 209.8817) (187.2743, 210.0411) (187.2682, 210.2007) (187.2631, 210.3605) (187.2591, 210.5206) (187.2563, 210.6809) (187.2544, 210.8415) (187.2537, 211.0023) (187.254, 211.1633) (187.2554, 211.3245) (187.2578, 211.4859) (187.2612, 211.6475) (187.2655, 211.8093) (187.2709, 211.9712) (187.2772, 212.1334) (187.2845, 212.2957) (187.2928, 212.4581) (187.302, 212.6207) (187.3121, 212.7835) (187.3232, 212.9464) (187.3353, 213.1095) (187.3482, 213.2727) (187.362, 213.436) (187.3768, 213.5995) (187.3924, 213.7631) (187.409, 213.9268) (187.4264, 214.0906) (187.4447, 214.2545) (187.4639, 214.4185) (187.484, 214.5826) (187.5049, 214.7468) (187.5266, 214.9111) (187.5492, 215.0755) (187.5727, 215.24) (187.597, 215.4046) (187.6222, 215.5692) (187.6481, 215.734) (187.6749, 215.8987) (187.7026, 216.0636) (187.731, 216.2285) (187.7602, 216.3935) (187.7903, 216.5585) (187.8212, 216.7236) (187.8528, 216.8887) (187.8788, 217.0208) (187.8986, 217.1199) (187.912, 217.186) (187.9188, 217.2191) knots 0 0 0 0 0 0 0.01428571 0.02857143 0.04285714 0.05714286 0.07142857 0.08571429 0.1 0.11428571 0.12857143 0.14285714 0.15714286 0.17142857 0.18571429 0.2 0.21428571 0.22857143 0.24285714 0.25714286 0.27142857 0.28571429 0.3 0.31428571 0.32857143 0.34285714 0.35714286 0.37142857 0.38571429 0.4 0.41428571 0.42857143 0.44285714 0.45714286 0.47142857 0.48571429 0.5 0.51428571 0.52857143 0.54285714 0.55714286 0.57142857 0.58571429 0.6 0.61428571 0.62857143 0.64285714 0.65714286 0.67142857 0.68571429 0.7 0.71428571 0.72857143 0.74285714 0.75714286 0.77142857 0.78571429 0.8 0.81428571 0.82857143 0.84285714 0.85714286 0.87142857 0.88571429 0.9 0.91428571 0.92857143 0.94285714 0.95714286 0.97142857 0.98571429 1 1 1 1 1 1
  line L3172 (187.9372, 206.0345) -> (187.9249, 206.0628) construction
  line L3173 (187.9249, 206.0628) -> (187.9012, 206.1198) construction
  line L3174 (187.9012, 206.1198) -> (187.868, 206.2062) construction
  line L3175 (187.868, 206.2062) -> (187.8281, 206.3229) construction
  line L3176 (187.8281, 206.3229) -> (187.7842, 206.4711) construction
  line L3177 (187.7842, 206.4711) -> (187.7447, 206.6208) construction
  line L3178 (187.7447, 206.6208) -> (187.7079, 206.7714) construction
  line L3179 (187.7079, 206.7714) -> (187.6725, 206.9226) construction
  line L3180 (187.6725, 206.9226) -> (187.638, 207.0741) construction
  line L3181 (187.638, 207.0741) -> (187.6046, 207.226) construction
  line L3182 (187.6046, 207.226) -> (187.5726, 207.3783) construction
  line L3183 (187.5726, 207.3783) -> (187.5424, 207.5312) construction
  line L3184 (187.5424, 207.5312) -> (187.5144, 207.6848) construction
  line L3185 (187.5144, 207.6848) -> (187.4885, 207.8391) construction
  line L3186 (187.4885, 207.8391) -> (187.4646, 207.994) construction
  line L3187 (187.4646, 207.994) -> (187.4423, 208.1494) construction
  line L3188 (187.4423, 208.1494) -> (187.4215, 208.3052) construction
  line L3189 (187.4215, 208.3052) -> (187.4019, 208.4614) construction
  line L3190 (187.4019, 208.4614) -> (187.3835, 208.6179) construction
  line L3191 (187.3835, 208.6179) -> (187.3662, 208.7747) construction
  line L3192 (187.3662, 208.7747) -> (187.3502, 208.9318) construction
  line L3193 (187.3502, 208.9318) -> (187.3355, 209.0893) construction
  line L3194 (187.3355, 209.0893) -> (187.3222, 209.2471) construction
  line L3195 (187.3222, 209.2471) -> (187.3102, 209.4053) construction
  line L3196 (187.3102, 209.4053) -> (187.2995, 209.5638) construction
  line L3197 (187.2995, 209.5638) -> (187.29, 209.7226) construction
  line L3198 (187.29, 209.7226) -> (187.2816, 209.8817) construction
  line L3199 (187.2816, 209.8817) -> (187.2743, 210.0411) construction
  line L3200 (187.2743, 210.0411) -> (187.2682, 210.2007) construction
  line L3201 (187.2682, 210.2007) -> (187.2631, 210.3605) construction
  line L3202 (187.2631, 210.3605) -> (187.2591, 210.5206) construction
  line L3203 (187.2591, 210.5206) -> (187.2563, 210.6809) construction
  line L3204 (187.2563, 210.6809) -> (187.2544, 210.8415) construction
  line L3205 (187.2544, 210.8415) -> (187.2537, 211.0023) construction
  line L3206 (187.2537, 211.0023) -> (187.254, 211.1633) construction
  line L3207 (187.254, 211.1633) -> (187.2554, 211.3245) construction
  line L3208 (187.2554, 211.3245) -> (187.2578, 211.4859) construction
  line L3209 (187.2578, 211.4859) -> (187.2612, 211.6475) construction
  line L3210 (187.2612, 211.6475) -> (187.2655, 211.8093) construction
  line L3211 (187.2655, 211.8093) -> (187.2709, 211.9712) construction
  line L3212 (187.2709, 211.9712) -> (187.2772, 212.1334) construction
  line L3213 (187.2772, 212.1334) -> (187.2845, 212.2957) construction
  line L3214 (187.2845, 212.2957) -> (187.2928, 212.4581) construction
  line L3215 (187.2928, 212.4581) -> (187.302, 212.6207) construction
  line L3216 (187.302, 212.6207) -> (187.3121, 212.7835) construction
  line L3217 (187.3121, 212.7835) -> (187.3232, 212.9464) construction
  line L3218 (187.3232, 212.9464) -> (187.3353, 213.1095) construction
  line L3219 (187.3353, 213.1095) -> (187.3482, 213.2727) construction
  line L3220 (187.3482, 213.2727) -> (187.362, 213.436) construction
  line L3221 (187.362, 213.436) -> (187.3768, 213.5995) construction
  line L3222 (187.3768, 213.5995) -> (187.3924, 213.7631) construction
  line L3223 (187.3924, 213.7631) -> (187.409, 213.9268) construction
  line L3224 (187.409, 213.9268) -> (187.4264, 214.0906) construction
  line L3225 (187.4264, 214.0906) -> (187.4447, 214.2545) construction
  line L3226 (187.4447, 214.2545) -> (187.4639, 214.4185) construction
  line L3227 (187.4639, 214.4185) -> (187.484, 214.5826) construction
  line L3228 (187.484, 214.5826) -> (187.5049, 214.7468) construction
  line L3229 (187.5049, 214.7468) -> (187.5266, 214.9111) construction
  line L3230 (187.5266, 214.9111) -> (187.5492, 215.0755) construction
  line L3231 (187.5492, 215.0755) -> (187.5727, 215.24) construction
  line L3232 (187.5727, 215.24) -> (187.597, 215.4046) construction
  line L3233 (187.597, 215.4046) -> (187.6222, 215.5692) construction
  line L3234 (187.6222, 215.5692) -> (187.6481, 215.734) construction
  line L3235 (187.6481, 215.734) -> (187.6749, 215.8987) construction
  line L3236 (187.6749, 215.8987) -> (187.7026, 216.0636) construction
  line L3237 (187.7026, 216.0636) -> (187.731, 216.2285) construction
  line L3238 (187.731, 216.2285) -> (187.7602, 216.3935) construction
  line L3239 (187.7602, 216.3935) -> (187.7903, 216.5585) construction
  line L3240 (187.7903, 216.5585) -> (187.8212, 216.7236) construction
  line L3241 (187.8212, 216.7236) -> (187.8528, 216.8887) construction
  line L3242 (187.8528, 216.8887) -> (187.8788, 217.0208) construction
  line L3243 (187.8788, 217.0208) -> (187.8986, 217.1199) construction
  line L3244 (187.8986, 217.1199) -> (187.912, 217.186) construction
  line L3245 (187.912, 217.186) -> (187.9188, 217.2191) construction
  spline S43 degree 5 poles (187.9372, 206.0345) (187.9249, 206.0628) (187.9012, 206.1198) (187.868, 206.2062) (187.8281, 206.3229) (187.7842, 206.4711) (187.7447, 206.6208) (187.7079, 206.7714) (187.6725, 206.9226) (187.638, 207.0741) (187.6046, 207.226) (187.5726, 207.3783) (187.5424, 207.5312) (187.5144, 207.6848) (187.4885, 207.8391) (187.4646, 207.994) (187.4423, 208.1494) (187.4215, 208.3052) (187.4019, 208.4614) (187.3835, 208.6179) (187.3662, 208.7747) (187.3502, 208.9318) (187.3355, 209.0893) (187.3222, 209.2471) (187.3102, 209.4053) (187.2995, 209.5638) (187.29, 209.7226) (187.2816, 209.8817) (187.2743, 210.0411) (187.2682, 210.2007) (187.2631, 210.3605) (187.2591, 210.5206) (187.2563, 210.6809) (187.2544, 210.8415) (187.2537, 211.0023) (187.254, 211.1633) (187.2554, 211.3245) (187.2578, 211.4859) (187.2612, 211.6475) (187.2655, 211.8093) (187.2709, 211.9712) (187.2772, 212.1334) (187.2845, 212.2957) (187.2928, 212.4581) (187.302, 212.6207) (187.3121, 212.7835) (187.3232, 212.9464) (187.3353, 213.1095) (187.3482, 213.2727) (187.362, 213.436) (187.3768, 213.5995) (187.3924, 213.7631) (187.409, 213.9268) (187.4264, 214.0906) (187.4447, 214.2545) (187.4639, 214.4185) (187.484, 214.5826) (187.5049, 214.7468) (187.5266, 214.9111) (187.5492, 215.0755) (187.5727, 215.24) (187.597, 215.4046) (187.6222, 215.5692) (187.6481, 215.734) (187.6749, 215.8987) (187.7026, 216.0636) (187.731, 216.2285) (187.7602, 216.3935) (187.7903, 216.5585) (187.8212, 216.7236) (187.8528, 216.8887) (187.8788, 217.0208) (187.8986, 217.1199) (187.912, 217.186) (187.9188, 217.2191) knots 0 0 0 0 0 0 0.01428571 0.02857143 0.04285714 0.05714286 0.07142857 0.08571429 0.1 0.11428571 0.12857143 0.14285714 0.15714286 0.17142857 0.18571429 0.2 0.21428571 0.22857143 0.24285714 0.25714286 0.27142857 0.28571429 0.3 0.31428571 0.32857143 0.34285714 0.35714286 0.37142857 0.38571429 0.4 0.41428571 0.42857143 0.44285714 0.45714286 0.47142857 0.48571429 0.5 0.51428571 0.52857143 0.54285714 0.55714286 0.57142857 0.58571429 0.6 0.61428571 0.62857143 0.64285714 0.65714286 0.67142857 0.68571429 0.7 0.71428571 0.72857143 0.74285714 0.75714286 0.77142857 0.78571429 0.8 0.81428571 0.82857143 0.84285714 0.85714286 0.87142857 0.88571429 0.9 0.91428571 0.92857143 0.94285714 0.95714286 0.97142857 0.98571429 1 1 1 1 1 1
  line L3246 (187.9372, 206.0345) -> (187.9249, 206.0628) construction
  line L3247 (187.9249, 206.0628) -> (187.9012, 206.1198) construction
  line L3248 (187.9012, 206.1198) -> (187.868, 206.2062) construction
  line L3249 (187.868, 206.2062) -> (187.8281, 206.3229) construction
  line L3250 (187.8281, 206.3229) -> (187.7842, 206.4711) construction
  line L3251 (187.7842, 206.4711) -> (187.7447, 206.6208) construction
  line L3252 (187.7447, 206.6208) -> (187.7079, 206.7714) construction
  line L3253 (187.7079, 206.7714) -> (187.6725, 206.9226) construction
  line L3254 (187.6725, 206.9226) -> (187.638, 207.0741) construction
  line L3255 (187.638, 207.0741) -> (187.6046, 207.226) construction
  line L3256 (187.6046, 207.226) -> (187.5726, 207.3783) construction
  line L3257 (187.5726, 207.3783) -> (187.5424, 207.5312) construction
  line L3258 (187.5424, 207.5312) -> (187.5144, 207.6848) construction
  line L3259 (187.5144, 207.6848) -> (187.4885, 207.8391) construction
  line L3260 (187.4885, 207.8391) -> (187.4646, 207.994) construction
  line L3261 (187.4646, 207.994) -> (187.4423, 208.1494) construction
  line L3262 (187.4423, 208.1494) -> (187.4215, 208.3052) construction
  line L3263 (187.4215, 208.3052) -> (187.4019, 208.4614) construction
  line L3264 (187.4019, 208.4614) -> (187.3835, 208.6179) construction
  line L3265 (187.3835, 208.6179) -> (187.3662, 208.7747) construction
  line L3266 (187.3662, 208.7747) -> (187.3502, 208.9318) construction
  line L3267 (187.3502, 208.9318) -> (187.3355, 209.0893) construction
  line L3268 (187.3355, 209.0893) -> (187.3222, 209.2471) construction
  line L3269 (187.3222, 209.2471) -> (187.3102, 209.4053) construction
  line L3270 (187.3102, 209.4053) -> (187.2995, 209.5638) construction
  line L3271 (187.2995, 209.5638) -> (187.29, 209.7226) construction
  line L3272 (187.29, 209.7226) -> (187.2816, 209.8817) construction
  line L3273 (187.2816, 209.8817) -> (187.2743, 210.0411) construction
  line L3274 (187.2743, 210.0411) -> (187.2682, 210.2007) construction
  line L3275 (187.2682, 210.2007) -> (187.2631, 210.3605) construction
  line L3276 (187.2631, 210.3605) -> (187.2591, 210.5206) construction
  line L3277 (187.2591, 210.5206) -> (187.2563, 210.6809) construction
  line L3278 (187.2563, 210.6809) -> (187.2544, 210.8415) construction
  line L3279 (187.2544, 210.8415) -> (187.2537, 211.0023) construction
  line L3280 (187.2537, 211.0023) -> (187.254, 211.1633) construction
  line L3281 (187.254, 211.1633) -> (187.2554, 211.3245) construction
  line L3282 (187.2554, 211.3245) -> (187.2578, 211.4859) construction
  line L3283 (187.2578, 211.4859) -> (187.2612, 211.6475) construction
  line L3284 (187.2612, 211.6475) -> (187.2655, 211.8093) construction
  line L3285 (187.2655, 211.8093) -> (187.2709, 211.9712) construction
  line L3286 (187.2709, 211.9712) -> (187.2772, 212.1334) construction
  line L3287 (187.2772, 212.1334) -> (187.2845, 212.2957) construction
  line L3288 (187.2845, 212.2957) -> (187.2928, 212.4581) construction
  line L3289 (187.2928, 212.4581) -> (187.302, 212.6207) construction
  line L3290 (187.302, 212.6207) -> (187.3121, 212.7835) construction
  line L3291 (187.3121, 212.7835) -> (187.3232, 212.9464) construction
  line L3292 (187.3232, 212.9464) -> (187.3353, 213.1095) construction
  line L3293 (187.3353, 213.1095) -> (187.3482, 213.2727) construction
  line L3294 (187.3482, 213.2727) -> (187.362, 213.436) construction
  line L3295 (187.362, 213.436) -> (187.3768, 213.5995) construction
  line L3296 (187.3768, 213.5995) -> (187.3924, 213.7631) construction
  line L3297 (187.3924, 213.7631) -> (187.409, 213.9268) construction
  line L3298 (187.409, 213.9268) -> (187.4264, 214.0906) construction
  line L3299 (187.4264, 214.0906) -> (187.4447, 214.2545) construction
  line L3300 (187.4447, 214.2545) -> (187.4639, 214.4185) construction
  line L3301 (187.4639, 214.4185) -> (187.484, 214.5826) construction
  line L3302 (187.484, 214.5826) -> (187.5049, 214.7468) construction
  line L3303 (187.5049, 214.7468) -> (187.5266, 214.9111) construction
  line L3304 (187.5266, 214.9111) -> (187.5492, 215.0755) construction
  line L3305 (187.5492, 215.0755) -> (187.5727, 215.24) construction
  line L3306 (187.5727, 215.24) -> (187.597, 215.4046) construction
  line L3307 (187.597, 215.4046) -> (187.6222, 215.5692) construction
  line L3308 (187.6222, 215.5692) -> (187.6481, 215.734) construction
  line L3309 (187.6481, 215.734) -> (187.6749, 215.8987) construction
  line L3310 (187.6749, 215.8987) -> (187.7026, 216.0636) construction
  line L3311 (187.7026, 216.0636) -> (187.731, 216.2285) construction
  line L3312 (187.731, 216.2285) -> (187.7602, 216.3935) construction
  line L3313 (187.7602, 216.3935) -> (187.7903, 216.5585) construction
  line L3314 (187.7903, 216.5585) -> (187.8212, 216.7236) construction
  line L3315 (187.8212, 216.7236) -> (187.8528, 216.8887) construction